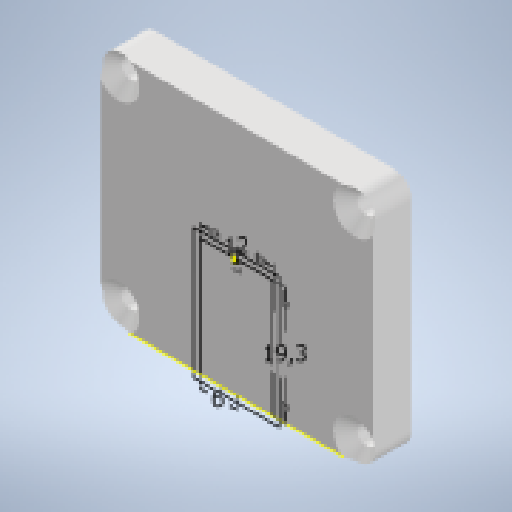
# Autodesk Inventor part: akkum_cap_bms
Saved by Autodesk Inventor 2025 (Build 290162000, 162)
## iProperties
Created: 2026-06-28
Part Number: akkum_cap_bms
Material: Типовые
Document SubType Name: Modeling
Designer: garin
Density: 1 g/cm^3
Appearance: По умолчанию
Author: garin
Autodesk Inventor part; units mm, degrees
ref_plane "YZ Plane" through (0, 0, 0) normal (1, 0, 0) x (0, 1, 0)
ref_plane "XZ Plane" through (0, 0, 0) normal (0, 1, 0) x (-1, 0, 0)
ref_plane "XY Plane" through (0, 0, 0) normal (0, 0, 1) x (1, 0, 0)
sketch "Эскиз1" plane through (0, 0, 0) normal (0, 0, 1) x (1, 0, 0)
  arc A0 (19.3, -19.3) -> (22.3, -16.3) centre (19.3, -16.3) ccw
  line L0 (19.3, -19.3) -> (-19.3, -19.3)
  arc A1 (-22.3, -16.3) -> (-19.3, -19.3) centre (-19.3, -16.3) ccw
  line L1 (-22.3, -16.3) -> (-22.3, 16.3)
  arc A2 (-19.3, 19.3) -> (-22.3, 16.3) centre (-19.3, 16.3) ccw
  line L2 (-19.3, 19.3) -> (19.3, 19.3)
  arc A3 (22.3, 16.3) -> (19.3, 19.3) centre (19.3, 16.3) ccw
  line L3 (22.3, 16.3) -> (22.3, -16.3)
  circle A4 centre (-19.3, 16.3) radius 2 construction
  circle A5 centre (19.3, 16.3) radius 2 construction
  circle A6 centre (19.3, -16.3) radius 2 construction
  circle A7 centre (-19.3, -16.3) radius 2 construction
  arc A8 (14.15, 1.4869) -> (1.4869, 14.15) centre (9.15, 9.15) ccw
  line L4 (1.4869, 14.15) -> (-1.4869, 14.15)
  arc A9 (-1.4869, 14.15) -> (-14.15, 1.4869) centre (-9.15, 9.15) ccw
  line L5 (-14.15, 1.4869) -> (-14.15, -1.4869)
  arc A10 (-14.15, -1.4869) -> (-1.4869, -14.15) centre (-9.15, -9.15) ccw
  line L6 (-1.4869, -14.15) -> (1.4869, -14.15)
  arc A11 (1.4869, -14.15) -> (14.15, -1.4869) centre (9.15, -9.15) ccw
  line L7 (14.15, -1.4869) -> (14.15, 1.4869)
  line L8 (-9.15, 9.15) -> (-18.3, 9.15) construction
  line L9 (-22.3, 0) -> (22.3, 0) construction
  line L10 (0, 19.3) -> (0, -19.3) construction
  line L11 (-9.15, -9.15) -> (-18.3, -9.15) construction
  line L12 (-9.15, 9.15) -> (-9.15, 18.3) construction
  line L13 (9.15, 9.15) -> (9.15, 18.3) construction
  line L14 (-18.3, 9.15) -> (-18.3, -9.15)
  line L15 (-9.15, 18.3) -> (9.15, 18.3)
  line L16 (-9.15, -18.3) -> (9.15, -18.3)
  line L17 (18.3, 9.15) -> (18.3, -9.15)
  line L18 (-18.3, 9.15) -> (-18.3, 4.15) construction
  line L19 (-18.3, -9.15) -> (-18.3, -4.15) construction
  line L20 (-18.3, 4.15) -> (-21.3, 4.15)
  line L21 (-21.3, 4.15) -> (-21.3, -4.15)
  line L22 (-21.3, -4.15) -> (-18.3, -4.15)
  line L23 (-18.3, -4.15) -> (-18.3, 4.15)
  line L24 (18.3, 4.15) -> (21.3, 4.15)
  line L25 (21.3, 4.15) -> (21.3, -4.15)
  line L26 (21.3, -4.15) -> (18.3, -4.15)
  line L27 (18.3, -4.15) -> (18.3, 4.15)
  circle A12 centre (-19.3, 16.3) radius 1.5
  circle A13 centre (19.3, 16.3) radius 1.5
  circle A14 centre (19.3, -16.3) radius 1.5
  circle A15 centre (-19.3, -16.3) radius 1.5
  dimension "d0" = 5
  dimension "d1" = 5
  dimension "d2" = 3
  dimension "d3" = 8.3
  dimension "d4" = 3
  dimension "d5" = 3
  dimension "d6" = 3
  dimension "d7" = 3
  constraints: 56 end point, 20 point on circle, 16 centre point, 8 symmetric about line, 7 horizontal, 7 vertical, 4 coincident, 4 midpoint, 3 parallel, 2 point on line, 1 perpendicular, 1 tangent, 40 other
  measures "d0" distance of L8.end L18.end
  measures "d1" distance of L11.end L19.end
  measures "d2" distance of L22.end L21.end
  measures "d3" distance of L21.end L20.end
  measures "d4" diameter of A12
  measures "d5" diameter of A13
  measures "d6" diameter of A14
  measures "d7" diameter of A15
extrude "Выдавливание1" add sketch "Эскиз1" along normal blind 6.4 contours L0 A1 L1 A2 L2 A3 L3 A0 | L7 A11 L6 A10 L5 A9 L4 A8 | A8 L17 A11 L7 | A8 L4 A9 L15 | L24 L25 L26 L17 | L16 A10 L6 A11 | A9 L5 A10 L14 | L14 L22 L21 L20
extrude "Выдавливание2" cut sketch "Эскиз1" along normal blind 5.4 contours L7 A11 L6 A10 L5 A9 L4 A8 | A8 L17 A11 L7 | A8 L4 A9 L15 | L24 L25 L26 L17 | L16 A10 L6 A11 | A9 L5 A10 L14 | L14 L22 L21 L20
chamfer "Фаска1" distance 2 angle 45 4 edges at (17.8, 16.3, 6.4) (17.8, -16.3, 6.4) (-20.8, -16.3, 6.4) (-20.8, 16.3, 6.4)
fillet "Сопряжение1" radius 2 2 edges at (-21.3, 0, 5.4) (21.3, 0, 5.4)
sketch "Эскиз2" plane through (0, 0, 6.4) normal (0, 0, 1) x (1, 0, 0)
  line L0 (-17.4972, -19.3) -> (17.4972, -19.3) projected
  line L1 (0, -19.3) -> (-6, -19.3)
  line L2 (-6, -19.3) -> (6, -19.3)
  line L3 (6, -19.3) -> (6, 0)
  line L4 (6, 0) -> (-6, 0)
  line L5 (-6, 0) -> (-6, -19.3)
  line L6 (-7, 1) -> (7, 1)
  line L7 (7, 1) -> (7, -20.3)
  line L8 (7, -20.3) -> (-7, -20.3)
  line L9 (-7, -20.3) -> (-7, 1)
  line L10 (-6, -19.3) -> (6, -19.3)
  line L11 (6, -19.3) -> (6, -18.3)
  line L12 (6, -18.3) -> (-6, -18.3)
  line L13 (-6, -18.3) -> (-6, -19.3)
  line L14 (6, -18.3) -> (-6, -18.3)
  line L15 (-6, -18.3) -> (-6, -17.3)
  line L16 (-6, -17.3) -> (6, -17.3)
  line L17 (6, -17.3) -> (6, -18.3)
  line L18 (-6, -17.3) -> (6, -17.3)
  line L19 (6, -17.3) -> (6, -16.3)
  line L20 (6, -16.3) -> (-6, -16.3)
  line L21 (-6, -16.3) -> (-6, -17.3)
  line L22 (-6, -16.3) -> (6, -16.3)
  line L23 (6, -16.3) -> (6, -15.3)
  line L24 (6, -15.3) -> (-6, -15.3)
  line L25 (-6, -15.3) -> (-6, -16.3)
  line L26 (-6, 0) -> (-6, 1)
  line L27 (6, 0) -> (6, 1)
  point P0 (0, 0)
  point P1 (7, -19.3)
  point P2 (-7, -19.3)
  dimension "d16" = 6
  dimension "d17" = 12
  dimension "d18" = 19.3
  dimension "d19" = 1
  dimension "d20" = 1
  dimension "d21" = 1
  dimension "d22" = 12
  dimension "d23" = 1
  dimension "d24" = 1
  constraints: 54 end point, 12 parallel, 8 perpendicular, 6 point on line, 5 horizontal, 1 midpoint, 3 other
  measures "d16" distance of L1.start L1.end
  measures "d17" distance of L4.end L3.end
  measures "d18" distance of L3.end L2.end
  measures "d19" distance between parallel lines of L4 L6
  measures "d20" distance of L11.end L10.end
  measures "d21" distance of L14.end L15.end
  measures "d22" distance of L20.end L19.end
  measures "d23" distance of L19.end L18.end
  measures "d24" distance of L23.end L22.end
extrude "Выдавливание3" cut sketch "Эскиз2" against normal blind 10 contours L0 L9 L6 L26 L5 | L3 L27 L6 L7 L0
extrude "Выдавливание4" cut sketch "Эскиз2" against normal blind 0.4 contours L5 L16 L3 L12 | L5 L24 L3 L20
ref_plane "РабПлоскость1" through (0, -16.3, 0) normal (-1, 0, 0) x (0, 0, 1)
sketch "Эскиз3" plane through (0, -16.3, 0) normal (-1, 0, 0) x (0, 0, 1)
  line L0 (0, -3) -> (6.4, -3) projected
  line L1 (6.4, -3) -> (6.4, 1)
  line L2 (6.4, -3) -> (6.4, 3.5) projected
  line L3 (6.4, 1) -> (6.4, -2)
  point P0 (0, 16.3)
  point P1 (6.4, 1.8028)
  dimension "d29" = 4
  dimension "d30" = 3
  constraints: 4 end point, 2 point on line
  measures "d29" distance of L0.end L1.end
  measures "d30" distance of L1.end L3.end
sketch "Эскиз5" plane through (6, -18.3, 5.4) normal (1, 0, 0) x (0, 0, -1)
  line L0 (-1, 5.5) -> (-1, -1) projected
  line L1 (-1, -1) -> (-1, 3)
  line L2 (-1, 3) -> (-4, 3)
  line L3 (-1, 3) -> (-1, 6)
  line L4 (-1, 6) -> (-4, 3)
  line L5 (-1, 3) -> (-3, 3)
  line L6 (-3, 3) -> (-3, 4)
  line L7 (-3, 4) -> (-1, 4)
  line L8 (-1, 4) -> (-1, 3)
  line L9 (-3, 4) -> (-2.4226, 3)
  line L10 (-3, 4) -> (-1.8453, 4) construction
  point P0 (5.4, 18.3)
  point P1 (-1, 3.8028)
  point P2 (-2.4226, 3)
  dimension "d31" = 4
  dimension "d32" = 3
  dimension "d33" = 3
  dimension "d34" = 2
  dimension "d35" = 60
  constraints: 20 end point, 4 point on line, 3 horizontal, 2 parallel, 1 equal length, 1 perpendicular
  measures "d31" distance of L0.end L1.end
  measures "d32" distance of L1.end L2.end
  measures "d33" distance of L1.end L3.end
  measures "d34" distance of L6.end L7.end
  measures "d35" angle of L9 L10
extrude "Выдавливание5" add sketch "Эскиз5" against normal blind 12 contours L0 L7 L4 L3 | L0 L2 L9 L7
sketch "Эскиз8" plane through (6, -18.3, 5.4) normal (1, 0, 0) x (0, 0, -1)
  point P0 (5.4, 18.3)
sketch "Эскиз9" plane through (-6, -19.3, 0) normal (0, -1, 0) x (1, 0, 0)
  line L0 (12, 5.4) -> (12, 0) projected
  line L1 (12, 0) -> (0, 0)
  line L2 (0, 0) -> (0, 4.4)
  line L3 (0, 4.4) -> (12, 4.4)
  line L4 (12, 4.4) -> (12, 0)
  line L5 (0, 4.4) -> (12, 4.4)
  line L6 (12, 4.4) -> (12, 5.4)
  line L7 (12, 5.4) -> (0, 5.4)
  line L8 (0, 5.4) -> (0, 4.4)
  point P0 (6, 0)
  dimension "d38" = 12
  dimension "d39" = 4.4
  constraints: 16 end point, 4 parallel, 2 horizontal, 2 perpendicular
  measures "d38" distance of L2.end L3.end
  measures "d39" distance of L1.end L2.end
extrude "Выдавливание6" cut sketch "Эскиз9" against normal blind 12
sketch "Эскиз4" plane through (6, -18.3, 5.4) normal (1, 0, 0) x (0, 0, -1)
  point P0 (5.4, 18.3)
